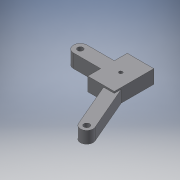
# Autodesk Inventor part: tiller frame bracket
Saved by Autodesk Inventor 2017 (Build 210142000, 142)
## iProperties
Created: 2017-12-08
Part Number: tiller frame bracket
Material: Generic
Document SubType Name: Modeling
Designer: RLanting
Density: 1 g/cm^3
Appearance: Default
Author: RLanting
Autodesk Inventor part; units mm, degrees
ref_plane "YZ Plane" through (0, 0, 0) normal (1, 0, 0) x (0, 1, 0)
ref_plane "XZ Plane" through (0, 0, 0) normal (0, 1, 0) x (-1, 0, 0)
ref_plane "XY Plane" through (0, 0, 0) normal (0, 0, 1) x (1, 0, 0)
sketch "Sketch1" plane through (0, 0, 0) normal (0, 0, 1) x (1, 0, 0)
  line L0 (9.525, -19.05) -> (-9.525, -19.05)
  line L1 (-9.525, -19.05) -> (-9.525, 19.05)
  line L2 (-9.525, 19.05) -> (9.525, 19.05)
  line L3 (9.525, 19.05) -> (9.525, -19.05)
  line L4 (9.525, -19.05) -> (-9.525, 19.05) construction
  line L5 (-9.525, -19.05) -> (9.525, 19.05) construction
  line L6 (19.525, -29.05) -> (-19.525, -29.05)
  line L7 (-19.525, -29.05) -> (-19.525, 29.05)
  line L8 (-19.525, 29.05) -> (19.525, 29.05)
  line L9 (19.525, 29.05) -> (19.525, -29.05)
  line L10 (19.525, -29.05) -> (-19.525, 29.05) construction
  line L11 (-19.525, -29.05) -> (19.525, 29.05) construction
  line L12 (-19.525, 0) -> (-59.525, 0) construction
  circle A0 centre (-59.525, 0) radius 4
  line L13 (-59.525, 0) -> (-19.525, 0) construction
  line L14 (-59.525, -10) -> (-19.525, -10)
  line L15 (-19.525, 10) -> (-59.525, 10)
  arc A1 (-59.525, 10) -> (-59.525, -10) centre (-59.525, 0) ccw
  arc A2 (-19.525, -10) -> (-19.525, 10) centre (-19.525, 0) ccw construction
  line L16 (-19.525, 10) -> (-19.525, -10)
  point P0 (0, 0)
  point P1 (-39.525, 0)
  dimension "d0" = 38.1
  dimension "d1" = 19.05
  dimension "d2" = 10
  dimension "d3" = 10
  dimension "d4" = 8
  dimension "d5" = 10
  dimension "d6" = 40
  constraints: 36 end point, 6 midpoint, 5 parallel, 4 horizontal, 4 point on circle, 4 tangent, 3 centre point, 2 perpendicular, 1 coincident, 1 collinear
  measures "d0" distance of L0.end L1.end
  measures "d1" distance of L1.end L2.end
  measures "d2" distance between parallel lines of L1 L7
  measures "d3" distance between parallel lines of L2 L8
  measures "d4" diameter of A0
  measures "d5" radius of A1
  measures "d6" distance of L13.start L12.start
extrude "Extrusion1" add sketch "Sketch1" along normal blind 15
sketch "Sketch2" plane through (0, 0, 15) normal (0, 0, 1) x (1, 0, 0)
  line L0 (-9.525, -19.05) -> (-9.525, 19.05) projected
  line L1 (-9.525, 19.05) -> (9.525, 19.05) projected
  line L2 (9.525, 19.05) -> (9.525, -19.05) projected
  line L3 (9.525, -19.05) -> (-9.525, -19.05) projected
  circle A0 centre (-59.525, 0) radius 4 projected
  line L4 (-59.525, -10) -> (-19.525, -10) projected
  line L5 (-19.525, -10) -> (-19.525, -29.05) projected
  line L6 (-19.525, -29.05) -> (19.525, -29.05) projected
  line L7 (19.525, -29.05) -> (19.525, 29.05) projected
  line L8 (19.525, 29.05) -> (-19.525, 29.05) projected
  line L9 (-19.525, 29.05) -> (-19.525, 10) projected
  line L10 (-19.525, 10) -> (-59.525, 10) projected
  arc A1 (-59.525, 10) -> (-59.525, -10) centre (-59.525, 0) ccw projected
  point P0 (0, 0)
extrude "Extrusion2" add sketch "Sketch2" along normal blind 5 contours L0 L1 L2 L3 | A1 L10 L9 L8 L7 L6 L5 L4
sketch "Sketch3" plane through (0, 0, 15) normal (0, 0, -1) x (-1, 0, 0)
  circle A0 centre (0, 0) radius 2.5
  dimension "d11" = 5
  constraints: 1 centre point, 1 coincident
  measures "d11" diameter of A0
extrude "Extrusion3" cut sketch "Sketch3" against normal through all
sketch "Sketch4" plane through (0, 0, 20) normal (0, 0, 1) x (1, 0, 0)
  line L0 (0, 0) -> (40, 0) construction
  line L1 (40, 0) -> (40, -80) construction
  line L2 (40, -80) -> (0, -80) construction
  line L3 (0, -80) -> (0, 0) construction
  circle A0 centre (40, -80) radius 4.25
  line L4 (19.525, -29.05) -> (-19.525, -29.05) construction
  line L5 (19.525, -29.05) -> (9.525, -29.05) construction
  line L6 (9.525, -29.05) -> (9.525, -19.05) construction
  line L7 (9.525, -19.05) -> (19.525, -19.05) construction
  line L8 (19.525, -19.05) -> (19.525, -29.05) construction
  line L9 (9.525, -19.05) -> (40, -80) construction
  line L10 (1.2515, -23.1867) -> (31.7265, -84.1367)
  line L11 (48.2735, -75.8633) -> (17.7985, -14.9133)
  arc A1 (17.7985, -14.9133) -> (1.2515, -23.1867) centre (9.525, -19.05) ccw
  arc A2 (31.7265, -84.1367) -> (48.2735, -75.8633) centre (40, -80) ccw
  point P0 (24.7625, -49.525)
  dimension "d14" = 80
  dimension "d15" = 40
  dimension "d16" = 8.5
  dimension "d17" = 10
  dimension "d18" = 10
  dimension "d19" = 5
  constraints: 24 end point, 5 parallel, 4 point on circle, 4 tangent, 3 centre point, 2 horizontal, 2 perpendicular, 1 coincident, 1 midpoint
  measures "d14" distance of L0.end L1.end
  measures "d15" distance of L1.end L2.end
  measures "d16" diameter of A0
  measures "d17" distance of L6.end L7.end
  measures "d18" distance of L5.end L6.end
  measures "d19" radial gap between concentric circles of A0 A2
ref_plane "Work Plane1" through (26.995, -107.2374, 17.5) normal (0, 0, -1) x (0.0783612, 0.996925, 0)
extrude "Extrusion4" add sketch "Sketch4" along normal up to surface (17.5 mm away) from surface at -20
body "Solid1"
